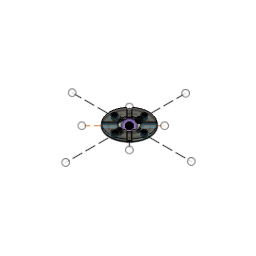
sphere_tray_disk v4 (Autodesk Fusion 360 design; units mm, degrees)
Autodesk Fusion 360 part; units mm, degrees
sketch "Skizze1" plane through (0, 0, 0) normal (0, 0, 1) x (1, 0, 0)
  line L0 (-52.7529, 0) -> (57.0438, 0) construction
  line L1 (0, 51.8694) -> (0, -58.6844) construction
  circle A0 centre (0, 0) radius 7.65
  circle A1 centre (0, 0) radius 18
  circle A2 centre (0, 0) radius 9.2 construction
  circle A3 centre (0, 9.2) radius 1.2
  circle A4 centre (0, -9.2) radius 1.2
  line L2 (-14.9273, 14.9273) -> (19.3405, -19.3405) construction
  line L3 (16.2492, 16.2492) -> (-21.9212, -21.9212) construction
  circle A5 centre (0, 0) radius 13.642 construction
  line L4 (-1.3279, 15.942) -> (-2.6558, 13.642)
  line L5 (-2.6558, 13.642) -> (-1.3279, 11.342)
  line L6 (-1.3279, 11.342) -> (1.3279, 11.342)
  line L7 (1.3279, 11.342) -> (2.6558, 13.642)
  line L8 (2.6558, 13.642) -> (1.3279, 15.942)
  line L9 (1.3279, 15.942) -> (-1.3279, 15.942)
  line L10 (-15.942, -1.3279) -> (-13.642, -2.6558)
  line L11 (-13.642, -2.6558) -> (-11.342, -1.3279)
  line L12 (-11.342, -1.3279) -> (-11.342, 1.3279)
  line L13 (-11.342, 1.3279) -> (-13.642, 2.6558)
  line L14 (-13.642, 2.6558) -> (-15.942, 1.3279)
  line L15 (-15.942, 1.3279) -> (-15.942, -1.3279)
  line L16 (1.3279, -15.942) -> (2.6558, -13.642)
  line L17 (2.6558, -13.642) -> (1.3279, -11.342)
  line L18 (1.3279, -11.342) -> (-1.3279, -11.342)
  line L19 (-1.3279, -11.342) -> (-2.6558, -13.642)
  line L20 (-2.6558, -13.642) -> (-1.3279, -15.942)
  line L21 (-1.3279, -15.942) -> (1.3279, -15.942)
  line L22 (15.942, 1.3279) -> (13.642, 2.6558)
  line L23 (13.642, 2.6558) -> (11.342, 1.3279)
  line L24 (11.342, 1.3279) -> (11.342, -1.3279)
  line L25 (11.342, -1.3279) -> (13.642, -2.6558)
  line L26 (13.642, -2.6558) -> (15.942, -1.3279)
  line L27 (15.942, -1.3279) -> (15.942, 1.3279)
  line L28 (-9.5, 1) -> (-7.5844, 1)
  line L29 (-9.5, -1) -> (-7.5844, -1)
  line L30 (-9.5, 1) -> (-9.5, -1)
  line L31 (9.5, 1) -> (9.5, -1)
  line L32 (7.5844, -1) -> (9.5, -1)
  line L33 (7.5844, 1) -> (9.5, 1)
  line L34 (-6.365, -4.2437) -> (-13.7443, -11.623)
  line L35 (-4.2437, -6.365) -> (-11.623, -13.7443)
  line L36 (-11.623, 13.7443) -> (-4.2437, 6.365)
  line L37 (-13.7443, 11.623) -> (-6.365, 4.2437)
  line L38 (11.623, 13.7443) -> (4.2437, 6.365)
  line L39 (13.7443, 11.623) -> (6.365, 4.2437)
  line L40 (6.365, -4.2437) -> (13.7443, -11.623)
  line L41 (4.2437, -6.365) -> (11.623, -13.7443)
  point P0 (0, 9.2)
  point P1 (0, -9.2)
  point P2 (0, -13.642)
  point P3 (-13.642, 0)
  point P4 (0, 13.642)
  point P5 (13.642, 0)
  point P6 (0, 13.642)
  point P7 (-13.642, 0)
  point P8 (0, -13.642)
  point P9 (13.642, 0)
  dimension "d1" = 15.3
  dimension "d3" = 36
  dimension "d4" = 18.4
  dimension "d5" = 2.4
  dimension "d6" = 2.4
  dimension "d7" = 45
  dimension "d8" = 45
  dimension "d17" = 27.284
  dimension "d18" = 4.6
  dimension "d19" = 4.6
  dimension "d20" = 4.6
  dimension "d21" = 4.6
  dimension "d26" = 1
  dimension "d27" = 1
  dimension "d28" = 9.5
  dimension "d29" = 9.5
  dimension "d30" = 1
  dimension "d31" = 1
  dimension "d32" = 1.5
  dimension "d33" = 1.5
  dimension "d34" = 1.5
  dimension "d35" = 1.5
  dimension "d36" = 1.5
  dimension "d37" = 1.5
  dimension "d38" = 1.5
  dimension "d39" = 1.5
  constraint horizontal L0
  constraint coincident A0.centre L0
  constraint vertical L1
  constraint coincident A0.centre L1
  constraint coincident A0.centre A1.centre
  constraint coincident A2 P0
  constraint coincident L1 P0
  constraint coincident A2 P1
  constraint coincident L1 P1
  constraint coincident P0 A3.centre
  constraint coincident P1 A4.centre
  constraint coincident A0.centre L2
  constraint coincident L1 P8
  constraint coincident A5 P8
  constraint coincident A5 P7
  constraint coincident L0 P7
  constraint coincident L1 P6
  constraint coincident A5 P6
  constraint coincident A5 P9
  constraint coincident L0 P9
  constraint coincident P6 P4
  constraint coincident P7 P3
  constraint coincident P8 P2
  constraint coincident P9 P5
  constraint horizontal L28
  constraint horizontal L29
  constraint coincident A0 L28.end
  constraint coincident A0 L29.end
  constraint perpendicular L28 L30
  constraint vertical L31
  constraint horizontal L32
  constraint horizontal L33
  constraint coincident A0 L33.start
  constraint coincident A0 L32.start
  constraint coincident L31 L33.end
  constraint coincident L31 L32.end
  constraint coincident L31.end L32
  constraint coincident L31.start L33
  constraint coincident L28 L30.start
  constraint coincident L28.start L30
  constraint coincident L29.start L30
  constraint coincident L29 L30.end
  constraint parallel L3 L35
  constraint parallel L3 L34
  constraint parallel L2 L37
  constraint parallel L2 L36
  constraint parallel L3 L38
  constraint parallel L3 L39
  constraint parallel L2 L40
  constraint parallel L2 L41
  constraint coincident A0 L40.start
  constraint coincident A0 L41.start
  constraint coincident A1 L41.end
  constraint coincident A1 L40.end
  constraint coincident A0 L39.end
  constraint coincident A0 L38.end
  constraint coincident A1 L38.start
  constraint coincident A1 L39.start
  constraint coincident A0 L36.end
  constraint coincident A0 L37.end
  constraint coincident A1 L37.start
  constraint coincident A1 L36.start
  constraint coincident A0 L34.start
  constraint coincident A0 L35.start
  constraint coincident A1 L35.end
  constraint coincident A1 L34.end
  measures "d1" diameter of A0
  measures "d3" diameter of A1
  measures "d4" diameter of A2
  measures "d5" diameter of A4
  measures "d6" diameter of A3
  measures "d7" angle of L0 L2
  measures "d8" angle of L0 L3
  measures "d17" diameter of A5
  measures "d18" distance of L24 L27
  measures "d19" distance of L18 L21
  measures "d20" distance of L12 L15
  measures "d21" distance of L6 L9
  measures "d26" distance of L0 L29
  measures "d27" distance of L0 L28
  measures "d28" distance of A0.centre L30
  measures "d29" distance of A0.centre L31
  measures "d30" distance of L0 L32
  measures "d31" distance of L0 L33
  measures "d32" distance of L3 L34
  measures "d33" distance of L3 L35
  measures "d34" distance of L2 L37
  measures "d35" distance of L2 L36
  measures "d36" distance of L3 L38
  measures "d37" distance of L3 L39
  measures "d38" distance of L2 L40
  measures "d39" distance of A0.centre L41
extrude "Extrusion1" add sketch "Skizze1" along normal blind 1 contours A0 A1 L31 L32 L33 L39 L40 | A0 A1 L38 L39 | A0 A1 L40 L41 | A0 A1 L36 L38 | A0 A1 L35 L41 | A0 A1 L36 L37 | A0 A1 L34 L35 | A0 A1 L28 L29 L30 L34 L37
extrude "Extrusion2" add sketch "Skizze1" along normal blind 2 contours A0 A1 L31 L32 L33 L39 L40 | A0 A1 L36 L38 | A0 A1 L35 L41 | A0 A1 L28 L29 L30 L34 L37
